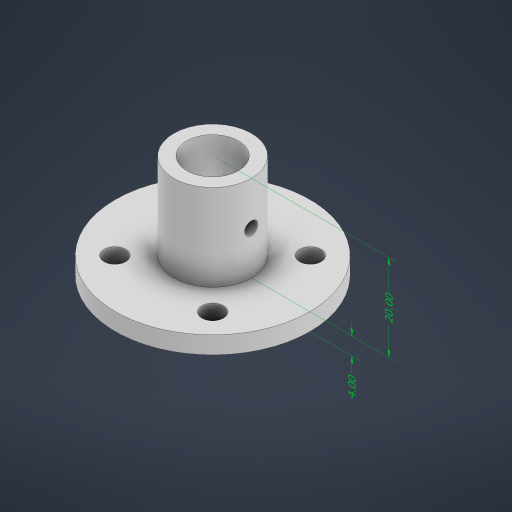
# Autodesk Inventor part: 12mm Flange
Saved by Autodesk Inventor 2023 (Build 270158000, 158)
## iProperties
Created: 2023-09-12
Part Number: 12mm Flange
Material: Generic
Document SubType Name: Modeling
Designer: Abhinav
Density: 1 g/cm^3
Appearance: Default
Author: Abhinav
Autodesk Inventor part; units mm, degrees
ref_plane "YZ Plane" through (0, 0, 0) normal (1, 0, 0) x (0, 1, 0)
ref_plane "XZ Plane" through (0, 0, 0) normal (0, 1, 0) x (-1, 0, 0)
ref_plane "XY Plane" through (0, 0, 0) normal (0, 0, 1) x (1, 0, 0)
sketch "Sketch1" plane through (0, 0, 0) normal (0, 1, 0) x (-1, 0, 0)
  circle A0 centre (0, 0) radius 6
  circle A1 centre (0, 0) radius 22.5
  circle A2 centre (0, 0) radius 9
  line L0 (0, 0) -> (11.3137, -11.3137) construction
  line L1 (0, 0) -> (16, 0) construction
  line L2 (0, 0) -> (-11.3137, 11.3137) construction
  circle A3 centre (11.3137, -11.3137) radius 2.5
  circle A4 centre (-11.3137, 11.3137) radius 2.5
  circle A5 centre (11.3137, 11.3137) radius 2.5
  circle A6 centre (-11.3137, -11.3137) radius 2.5
  dimension "d0" = 12
  dimension "d1" = 45
  dimension "d2" = 18
  dimension "d8" = 45
  dimension "d9" = 16
  dimension "d10" = 5
  constraints: 7 centre point, 6 end point, 5 coincident, 2 equal length, 2 symmetric about line, 1 equal radius, 1 horizontal, 2 other
  measures "d0" diameter of A0
  measures "d1" diameter of A1
  measures "d2" diameter of A2
  measures "d8" angle of L0 L1
  measures "d9" distance of L0.start L2.end
  measures "d10" diameter of A3
extrude "Extrusion1" add sketch "Sketch1" along normal blind 20 contours A2
extrude "Extrusion2" add sketch "Sketch1" against normal blind 4 contours A0 | A1 | A2
sketch "Sketch2" plane through (0, 0, 0) normal (1, 0, 0) x (0, 1, 0)
  line L0 (0, 0) -> (10, 0) construction
  circle A0 centre (10, 0) radius 1.5
  dimension "d12" = 10
  dimension "d13" = 3
  constraints: 2 end point, 1 centre point, 1 coincident, 1 horizontal
  measures "d12" distance of L0.start L0.end
  measures "d13" diameter of A0
extrude "Extrusion3" cut sketch "Sketch2" along normal mid plane 30
body "Solid1"
